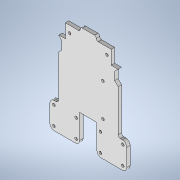
# Autodesk Inventor part: Основа робота
Saved by Autodesk Inventor 2020 (Build 240168000, 168)
## iProperties
Created: 2021-02-28
Part Number: Основа робота
Material: Типовые
Document SubType Name: Обычные детали
Designer: Антон
Density: 1 g/cm^3
Appearance: По умолчанию
Mass: 52.0111 g
Surface Area: 352.197 cm^2
Volume: 52.0111 cm^3
Sheet Metal Rule: По умолчанию
Author: Антон
Autodesk Inventor part; units mm, degrees
note: some values were not read from the file. Chosen so that the rebuilt part matches the saved one: direction of "Рельеф1".
ref_plane "YZ Plane" through (0, 0, 0) normal (1, 0, 0) x (0, 1, 0)
ref_plane "XZ Plane" through (0, 0, 0) normal (0, 1, 0) x (-1, 0, 0)
ref_plane "XY Plane" through (0, 0, 0) normal (0, 0, 1) x (1, 0, 0)
sketch "Эскиз1" plane through (0, 0, 0) normal (0, 0, 1) x (1, 0, 0)
  line L0 (0, 0) -> (34.5, 0)
  line L1 (34.5, 0) -> (34.5, 114.55)
  line L2 (34.5, 114.55) -> (0, 114.55)
  line L3 (0, 114.55) -> (0, 0)
  line L4 (0, 0) -> (-9.9, 0)
  line L5 (-9.9, 0) -> (-9.9, 30.3)
  line L6 (-9.9, 30.3) -> (0, 30.3)
  line L7 (0, 30.3) -> (0, 0)
  line L8 (-9.9, 0) -> (-5.35, 0)
  line L9 (-5.35, 0) -> (-5.35, 4.55)
  line L10 (-5.35, 4.55) -> (-5.35, 25.75)
  circle A0 centre (-5.35, 25.75) radius 1.6
  circle A1 centre (-5.35, 4.55) radius 1.6
  line L11 (34.5, 0) -> (24.5, 0)
  line L12 (24.5, 0) -> (24.5, 33)
  line L13 (24.5, 33) -> (34.5, 33)
  line L14 (34.5, 33) -> (34.5, 0)
  line L15 (24.5, 4.55) -> (20.5, 4.55)
  line L16 (24.5, 25.75) -> (20.5, 25.75)
  circle A2 centre (20.5, 25.75) radius 1.6
  circle A3 centre (20.5, 4.55) radius 1.6
  line L17 (34.5, 114.55) -> (34.5, 114.55)
  line L18 (34.5, 114.55) -> (18, 114.55)
  line L19 (20.5, 25.75) -> (20.5, 4.55)
  circle A4 centre (12.95, 106.55) radius 1.6
  line L20 (8, 114.55) -> (8, 98.55)
  line L21 (8, 98.55) -> (0, 98.55)
  line L22 (0, 98.55) -> (0, 129.6)
  line L23 (34.5, 114.55) -> (25.25, 114.55)
  line L24 (25.25, 114.55) -> (25.25, 119)
  line L25 (25.25, 119) -> (34.5, 119)
  line L26 (34.5, 119) -> (34.5, 114.55)
  line L27 (0, 98.55) -> (4, 94.55)
  line L28 (4, 94.55) -> (4, 85.125)
  line L29 (4, 85.125) -> (0, 81.125)
  point P0 (0, 30.3)
  point P1 (34.5, 33)
  point P2 (0, 182.1)
  point P3 (20.5, 15.15)
  point P4 (-5.35, 15.15)
  point P5 (0, 98.55)
  point P6 (8, 106.55)
  point P7 (0, 114.55)
  dimension "d0" = 34.5
  dimension "d1" = 114.55
  dimension "d191" = 9.9
  dimension "d192" = 30.3
  dimension "d207" = 4.55
  dimension "d208" = 4.55
  dimension "d209" = 21.2
  dimension "d210" = 10
  dimension "d211" = 33
  dimension "d215" = 4
  dimension "d290" = 3.2
  dimension "d387" = 21.2
  dimension "d418" = 4.55
  dimension "d421" = 3.2
  dimension "d427" = 8
  dimension "d428" = 16
  dimension "d433" = 4.95
  dimension "d448" = 9.25
  dimension "d450" = 4.45
  dimension "d453" = 45
  dimension "d454" = 4
  dimension "d455" = 17.425
  constraints: 60 end point, 10 parallel, 8 perpendicular, 8 point on line, 6 horizontal, 5 centre point, 4 coincident, 3 equal radius, 3 midpoint, 2 collinear, 2 horizontal alignment, 2 vertical
  measures "d0" distance of L2.end L1.end
  measures "d1" distance of L1.end L0.end
  measures "d191" distance of L5.end L6.end
  measures "d192" distance of L4.end L5.end
  measures "d207" distance of L4.end L8.end
  measures "d208" distance of L8.end L9.end
  measures "d209" distance of L9.end L10.end
  measures "d210" distance of L12.end L13.end
  measures "d211" distance of L11.end L12.end
  measures "d215" distance of L16.start L16.end
  measures "d290" diameter of A2
  measures "d387" distance of L19.end L19.start
  measures "d418" distance from line of L0 L15.end
  measures "d421" diameter of A4
  measures "d427" distance of L20.end L21.end
  measures "d428" distance of L20.start L20.end
  measures "d433" distance of A4.centre point (8, 106.55)
  measures "d448" distance of L24.end L25.end
  measures "d450" distance of L23.end L24.end
  measures "d453" angle of L3 L29
  measures "d454" distance between parallel lines of L3 L28
  measures "d455" distance of L21.end L29.end
extrude "Выдавливание1" add sketch "Эскиз1" along normal blind 4 contours L3 L29 L28 L27 L21 L20 L2 L1 L13 L12 L16 A2 L19 A3 L15 L0 | L4 L5 L6 L3 | L15 A3 L19 A2 L16 L12 | L2 L24 L25 L26
mirror "Зеркальное отражение1" about plane through (34.5, 33, 0) normal (1, 0, 0)
sketch "Эскиз32" plane through (0, 0, 4) normal (0, 0, 1) x (1, 0, 0)
  line L0 (24.5, 33) -> (34.5, 33) construction
  line L1 (34.5, 33) -> (34.5, 39.862) construction
  line L2 (34.5, 39.862) -> (51.4, 39.862) construction
  line L3 (51.4, 39.862) -> (51.4, 78.087) construction
  point P0 (0, 0)
  point P1 (44.5, 33)
  dimension "d434" = 6.862
  dimension "d435" = 16.9
  dimension "d451" = 38.225
  constraints: 7 end point, 2 vertical, 1 horizontal
  measures "d434" distance of L0.end L1.end
  measures "d435" distance of L1.end L2.end
  measures "d451" distance of L2.end L3.end
hole "Отверстие14" at (51.4, 39.862, 4) at (51.4, 78.087, 4) direction (0, 0, -1) diameter 3.2 end through all
fillet "Сопряжение13" radius 2.225 4 edges at (25.25, 114.55, 2) (25.25, 119, 2) (43.75, 114.55, 2) (43.75, 119, 2)
fillet "Сопряжение2" radius 5.05 6 edges at (-9.9, 30.3, 2) (-9.9, 0, 2) (24.5, 0, 2) (44.5, 0, 2) (78.9, 0, 2) (78.9, 30.3, 2)
sketch "Эскиз19" plane through (0, 0, 0) normal (0, 0, -1) x (-1, 0, 0)
  line L0 (-15.75, 108.1666) -> (-12.95, 109.7832)
  line L1 (-12.95, 109.7832) -> (-10.15, 108.1666)
  line L2 (-10.15, 108.1666) -> (-10.15, 104.9334)
  line L3 (-10.15, 104.9334) -> (-12.95, 103.3168)
  line L4 (-12.95, 103.3168) -> (-15.75, 104.9334)
  line L5 (-15.75, 104.9334) -> (-15.75, 108.1666)
  line L6 (0, 81.125) -> (0, 30.3) projected
  circle A0 centre (-12.95, 106.55) radius 1.6 projected
  point P0 (0, 139.6)
  point P1 (-78, 139.6)
  point P2 (-14, 129.6)
  point P3 (-64, 129.6)
  point P4 (0, 119.25)
  point P5 (0, 97.45)
  point P6 (0, 129.6)
  point P7 (-78, 129.6)
  point P8 (-8, 114.55)
  point P9 (-61, 114.55)
  dimension "d423" = 5.6
  constraints: 12 end point, 1 coincident, 1 parallel, 14 other
  measures "d423" distance between parallel lines of L2 L5
extrude "Выдавливание7" cut sketch "Эскиз19" against normal blind 2.6 contours L0 L1 L2 L3 L4 L5 | A0
fillet "Сопряжение12" radius 2.725 2 edges at (69, 30.3, 2) (0, 30.3, 2)
sketch "Эскиз25" plane through (0, 0, 0) normal (0, 0, -1) x (-1, 0, 0)
  circle A0 centre (-20.5, 25.75) radius 1.6 projected
  circle A1 centre (-20.5, 4.55) radius 1.6 projected
  circle A2 centre (5.35, 25.75) radius 1.6 projected
  circle A3 centre (5.35, 4.55) radius 1.6 projected
  circle A4 centre (-48.5, 25.75) radius 1.6 projected
  circle A5 centre (-48.5, 4.55) radius 1.6 projected
  circle A6 centre (-74.35, 4.55) radius 1.6 projected
  circle A7 centre (-74.35, 25.75) radius 1.6 projected
  circle A8 centre (-56.05, 106.55) radius 1.6 projected
  circle A9 centre (-56.05, 106.55) radius 1.6 projected
  circle A10 centre (-51.4, 39.862) radius 1.6 projected
  circle A11 centre (-51.4, 39.862) radius 1.6 projected
  circle A12 centre (-51.4, 78.087) radius 1.6 projected
  point P0 (0, 0)
  constraints: 11 coincident
pattern_sketch "Массив по эскизу1" of "Выдавливание7" from (12.95, 106.55, 0) copies at (20.5, 25.75, 0) at (20.5, 4.55, 0) at (-5.35, 25.75, 0) at (-5.35, 4.55, 0) at (48.5, 25.75, 0) at (48.5, 4.55, 0) at (74.35, 4.55, 0) at (74.35, 25.75, 0) at (56.05, 106.55, 0) at (51.4, 39.862, 0) at (51.4, 78.087, 0)
fillet "Сопряжение11" radius 0.2 1 edges at (0, 98.55, 2)
sketch "Эскиз31" plane through (0, 0, 0) normal (0, 0, -1) x (-1, 0, 0)
  line L0 (-69, 98.55) -> (0, 98.55) construction
  line L1 (0, 98.55) -> (0, 33) construction
  line L2 (0, 33) -> (-69, 33) construction
  line L3 (-69, 33) -> (-69, 98.55) construction
  line L4 (-61, 98.55) -> (-69, 98.55) projected
  line L5 (-69, 81.125) -> (-69, 30.3) projected
  line L6 (0, 81.125) -> (0, 30.3) projected
  line L7 (-24.5, 33) -> (-44.5, 33) projected
  spline S0 degree 2 poles (-41.2437, 69.856) (-41.3342, 68.8754) (-42.5914, 67.7842) (-43.6374, 67.7842) knots 0 0 0 1 2 2 2
  spline S1 degree 2 poles (-43.6374, 67.7842) (-44.3666, 67.7842) (-45.473, 68.4781) (-46.0764, 69.7504) (-46.0915, 70.5903) knots 0 0 0 1 2 3 3 3
  line L8 (-46.0915, 70.5903) -> (-46.0915, 71.1635)
  spline S2 degree 2 poles (-46.0915, 71.1635) (-46.0915, 72.0285) (-45.478, 73.341) (-44.3364, 74.0551) (-43.5871, 74.0551) knots 0 0 0 1 2 3 3 3
  spline S3 degree 2 poles (-43.5871, 74.0551) (-42.5763, 74.0551) (-41.3443, 72.9639) (-41.2437, 71.9581) knots 0 0 0 1 2 2 2
  line L9 (-41.2437, 71.9581) -> (-42.2998, 71.9581)
  spline S4 degree 2 poles (-42.2998, 71.9581) (-42.3752, 72.6169) (-42.9887, 73.2002) (-43.5871, 73.2002) knots 0 0 0 1 2 2 2
  spline S5 degree 2 poles (-43.5871, 73.2002) (-44.2761, 73.2002) (-45.0204, 72.1894) (-45.0254, 71.2088) knots 0 0 0 1 2 2 2
  line L10 (-45.0254, 71.2088) -> (-45.0254, 70.6707)
  spline S6 degree 2 poles (-45.0254, 70.6707) (-45.0254, 69.68) (-44.3214, 68.6391) (-43.6374, 68.6391) knots 0 0 0 1 2 2 2
  spline S7 degree 2 poles (-43.6374, 68.6391) (-43.0139, 68.6391) (-42.3852, 69.2023) (-42.2998, 69.856) knots 0 0 0 1 2 2 2
  line L11 (-42.2998, 69.856) -> (-41.2437, 69.856)
  spline S8 degree 2 poles (-37.6883, 67.8697) (-37.7537, 68.0004) (-37.804, 68.2921) knots 0 0 0 1 1 1
  spline S9 degree 2 poles (-37.804, 68.2921) (-38.2918, 67.7842) (-38.9958, 67.7842) knots 0 0 0 1 1 1
  spline S10 degree 2 poles (-38.9958, 67.7842) (-39.6747, 67.7842) (-40.5397, 68.5636) (-40.5397, 69.1369) knots 0 0 0 1 2 2 2
  spline S11 degree 2 poles (-40.5397, 69.1369) (-40.5397, 69.8661) (-39.4635, 70.6405) (-38.4627, 70.6405) knots 0 0 0 1 2 2 2
  line L12 (-38.4627, 70.6405) -> (-37.8392, 70.6405)
  line L13 (-37.8392, 70.6405) -> (-37.8392, 70.9373)
  spline S12 degree 2 poles (-37.8392, 70.9373) (-37.8392, 71.2893) (-38.2314, 71.7117) (-38.6337, 71.7117) knots 0 0 0 1 2 2 2
  spline S13 degree 2 poles (-38.6337, 71.7117) (-38.9807, 71.7117) (-39.4232, 71.3647) (-39.4232, 71.0982) knots 0 0 0 1 2 2 2
  line L14 (-39.4232, 71.0982) -> (-40.4441, 71.0982)
  spline S14 degree 2 poles (-40.4441, 71.0982) (-40.4441, 71.4703) (-39.9513, 72.119) (-39.0964, 72.4861) (-38.5734, 72.4861) knots 0 0 0 1 2 3 3 3
  spline S15 degree 2 poles (-38.5734, 72.4861) (-37.7788, 72.4861) (-36.8334, 71.6866) (-36.8183, 70.9624) knots 0 0 0 1 2 2 2
  line L15 (-36.8183, 70.9624) -> (-36.8183, 68.9157)
  spline S16 degree 2 poles (-36.8183, 68.9157) (-36.8183, 68.3072) (-36.6473, 67.9401) knots 0 0 0 1 1 1
  line L16 (-36.6473, 67.9401) -> (-36.6473, 67.8697)
  line L17 (-36.6473, 67.8697) -> (-37.6883, 67.8697)
  spline S17 degree 2 poles (-38.8047, 68.5988) (-38.503, 68.5988) (-37.9699, 68.8955) (-37.8392, 69.142) knots 0 0 0 1 2 2 2
  line L18 (-37.8392, 69.142) -> (-37.8392, 70.0019)
  line L19 (-37.8392, 70.0019) -> (-38.3873, 70.0019)
  spline S18 degree 2 poles (-38.3873, 70.0019) (-38.9505, 70.0019) (-39.5238, 69.6046) (-39.5238, 69.2425) knots 0 0 0 1 2 2 2
  spline S19 degree 2 poles (-39.5238, 69.2425) (-39.5238, 68.9509) (-39.1316, 68.5988) (-38.8047, 68.5988) knots 0 0 0 1 2 2 2
  line L20 (-34.8068, 72.4006) -> (-34.7766, 71.8776)
  spline S20 degree 2 poles (-34.7766, 71.8776) (-34.2787, 72.4861) (-33.459, 72.4861) knots 0 0 0 1 1 1
  spline S21 degree 2 poles (-33.459, 72.4861) (-32.0459, 72.4861) (-32.0208, 70.8668) knots 0 0 0 1 1 1
  line L21 (-32.0208, 70.8668) -> (-32.0208, 67.8697)
  line L22 (-32.0208, 67.8697) -> (-33.0366, 67.8697)
  line L23 (-33.0366, 67.8697) -> (-33.0366, 70.8065)
  spline S22 degree 2 poles (-33.0366, 70.8065) (-33.0366, 71.239) (-33.4087, 71.6513) (-33.8312, 71.6513) knots 0 0 0 1 2 2 2
  spline S23 degree 2 poles (-33.8312, 71.6513) (-34.4497, 71.6513) (-34.7514, 71.0931) knots 0 0 0 1 1 1
  line L24 (-34.7514, 71.0931) -> (-34.7514, 67.8697)
  line L25 (-34.7514, 67.8697) -> (-35.7673, 67.8697)
  line L26 (-35.7673, 67.8697) -> (-35.7673, 72.4006)
  line L27 (-35.7673, 72.4006) -> (-34.8068, 72.4006)
  spline S24 degree 2 poles (-31.1709, 70.1678) (-31.1709, 71.2189) (-30.2003, 72.4861) (-29.3806, 72.4861) knots 0 0 0 1 2 2 2
  spline S25 degree 2 poles (-29.3806, 72.4861) (-28.6615, 72.4861) (-28.219, 71.9833) knots 0 0 0 1 1 1
  line L28 (-28.219, 71.9833) -> (-28.219, 74.3066)
  line L29 (-28.219, 74.3066) -> (-27.1981, 74.3066)
  line L30 (-27.1981, 74.3066) -> (-27.1981, 67.8697)
  line L31 (-27.1981, 67.8697) -> (-28.1234, 67.8697)
  line L32 (-28.1234, 67.8697) -> (-28.1737, 68.3373)
  spline S26 degree 2 poles (-28.1737, 68.3373) (-28.6313, 67.7842) (-29.3907, 67.7842) knots 0 0 0 1 1 1
  spline S27 degree 2 poles (-29.3907, 67.7842) (-30.1852, 67.7842) (-31.1709, 69.0665) (-31.1709, 70.1678) knots 0 0 0 1 2 2 2
  spline S28 degree 2 poles (-30.1551, 70.0823) (-30.1551, 69.3884) (-29.622, 68.6139) (-29.1292, 68.6139) knots 0 0 0 1 2 2 2
  spline S29 degree 2 poles (-29.1292, 68.6139) (-28.5056, 68.6139) (-28.219, 69.1721) knots 0 0 0 1 1 1
  line L33 (-28.219, 69.1721) -> (-28.219, 71.1082)
  spline S30 degree 2 poles (-28.219, 71.1082) (-28.5006, 71.6513) (-29.1242, 71.6513) knots 0 0 0 1 1 1
  spline S31 degree 2 poles (-29.1242, 71.6513) (-29.617, 71.6513) (-30.1551, 70.8668) (-30.1551, 70.0823) knots 0 0 0 1 2 2 2
  line L34 (-24.5529, 69.328) -> (-23.6276, 72.4006)
  line L35 (-23.6276, 72.4006) -> (-22.5464, 72.4006)
  line L36 (-22.5464, 72.4006) -> (-24.3467, 67.1807)
  spline S32 degree 2 poles (-24.3467, 67.1807) (-24.7591, 66.0391) (-25.7548, 66.0391) knots 0 0 0 1 1 1
  spline S33 degree 2 poles (-25.7548, 66.0391) (-25.9761, 66.0391) (-26.2426, 66.1146) knots 0 0 0 1 1 1
  line L37 (-26.2426, 66.1146) -> (-26.2426, 66.9091)
  line L38 (-26.2426, 66.9091) -> (-26.0515, 66.8941)
  spline S34 degree 2 poles (-26.0515, 66.8941) (-25.6643, 66.8941) (-25.2771, 67.1757) (-25.1614, 67.5025) knots 0 0 0 1 2 2 2
  line L39 (-25.1614, 67.5025) -> (-25.0156, 67.8948)
  line L40 (-25.0156, 67.8948) -> (-26.6097, 72.4006)
  line L41 (-26.6097, 72.4006) -> (-25.5084, 72.4006)
  line L42 (-25.5084, 72.4006) -> (-24.5529, 69.328)
  line L43 (-40.5799, 58.6565) -> (-39.031, 63.4289)
  line L44 (-39.031, 63.4289) -> (-37.8643, 63.4289)
  line L45 (-37.8643, 63.4289) -> (-40.0619, 57.3289)
  line L46 (-40.0619, 57.3289) -> (-41.0878, 57.3289)
  line L47 (-41.0878, 57.3289) -> (-43.2754, 63.4289)
  line L48 (-43.2754, 63.4289) -> (-42.1137, 63.4289)
  line L49 (-42.1137, 63.4289) -> (-40.5799, 58.6565)
  line L50 (-34.5855, 57.3289) -> (-35.6013, 57.3289)
  line L51 (-35.6013, 57.3289) -> (-35.6013, 62.227)
  line L52 (-35.6013, 62.227) -> (-37.0949, 61.7191)
  line L53 (-37.0949, 61.7191) -> (-37.0949, 62.574)
  line L54 (-37.0949, 62.574) -> (-34.7162, 63.449)
  line L55 (-34.7162, 63.449) -> (-34.5855, 63.449)
  line L56 (-34.5855, 63.449) -> (-34.5855, 57.3289)
  spline S35 degree 2 poles (-31.7643, 58.4001) (-31.4827, 58.4001) (-31.1709, 58.0782) (-31.1709, 57.8368) knots 0 0 0 1 2 2 2
  spline S36 degree 2 poles (-31.1709, 57.8368) (-31.1709, 57.5954) (-31.4827, 57.2836) (-31.7643, 57.2836) knots 0 0 0 1 2 2 2
  spline S37 degree 2 poles (-31.7643, 57.2836) (-32.0359, 57.2836) (-32.3577, 57.5954) (-32.3577, 58.0782) (-32.0459, 58.4001) (-31.7643, 58.4001) knots 0 0 0 1 2 3 4 4 4
  spline S38 degree 2 poles (-26.0918, 59.8987) (-26.0918, 58.5811) (-27.0774, 57.2434) (-28.0832, 57.2434) knots 0 0 0 1 2 2 2
  spline S39 degree 2 poles (-28.0832, 57.2434) (-29.0739, 57.2434) (-30.0746, 58.5459) (-30.0847, 59.8232) knots 0 0 0 1 2 2 2
  line L57 (-30.0847, 59.8232) -> (-30.0847, 60.8843)
  spline S40 degree 2 poles (-30.0847, 60.8843) (-30.0847, 62.1968) (-29.104, 63.5144) (-28.0932, 63.5144) knots 0 0 0 1 2 2 2
  spline S41 degree 2 poles (-28.0932, 63.5144) (-27.0925, 63.5144) (-26.1068, 62.232) (-26.0918, 60.9547) knots 0 0 0 1 2 2 2
  line L58 (-26.0918, 60.9547) -> (-26.0918, 59.8987)
  spline S42 degree 2 poles (-27.1126, 61.0402) (-27.1126, 61.9001) (-27.5803, 62.6997) (-28.0932, 62.6997) knots 0 0 0 1 2 2 2
  spline S43 degree 2 poles (-28.0932, 62.6997) (-28.5911, 62.6997) (-29.0588, 61.9404) (-29.0739, 61.1357) knots 0 0 0 1 2 2 2
  line L59 (-29.0739, 61.1357) -> (-29.0739, 59.7528)
  spline S44 degree 2 poles (-29.0739, 59.7528) (-29.0739, 58.8979) (-28.5961, 58.0581) (-28.0832, 58.0581) knots 0 0 0 1 2 2 2
  spline S45 degree 2 poles (-28.0832, 58.0581) (-27.5954, 58.0581) (-27.1227, 58.8325) (-27.1126, 59.6623) knots 0 0 0 1 2 2 2
  line L60 (-27.1126, 59.6623) -> (-27.1126, 61.0402)
  point P0 (0, 0)
  point P1 (-69, 97.45)
  point P2 (-69, 32.99)
  point P3 (0, 97.45)
  point P4 (-34.5, 33)
  constraints: 3 collinear, 1 horizontal, 3 other
emboss "Рельеф1" sketch "Эскиз31" operation cut depth 0.5 direction (0, 0, 1)
equation "\"Радиус_гибки\" = Толщина"
equation "\"Ширина_просечки\" = Толщина"
equation "\"Глубина_просечки\" = 0.5 * Толщина"
equation "\"Размер_просечки\" = 4 * Толщина"
equation "\"Мин_остаток\" = 2 * Толщина"
equation "\"Радиус_перехода\" = Радиус_гибки"
equation "\"Радиус_Якоби\" = Толщина"
equation "\"Размер_зазора\" = Толщина"
equation "\"Гайка_М3_з\" = 5.6"
equation "\"d130\" = 5.6"
equation "\"Толщина\" = 0.5"
